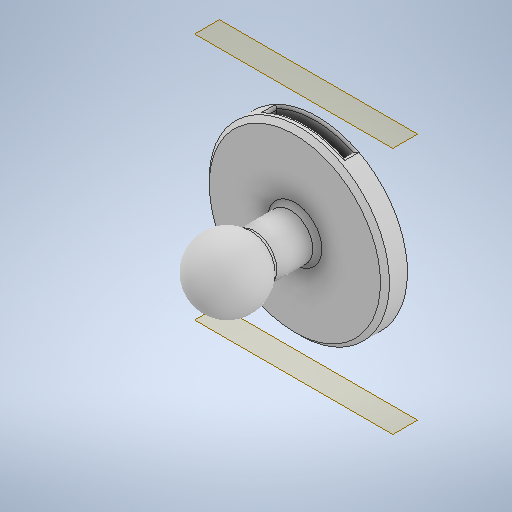
# Autodesk Inventor part: tagBase
Saved by Autodesk Inventor 2025 (Build 290162000, 162)
## iProperties
Created: 2026-08-22
Part Number: tagBase
Material: Generic
Document SubType Name: Modeling
Designer: PPSHS VR
Density: 1 g/cm^3
Appearance: Default
Author: PPSHS VR
Autodesk Inventor part; units mm, degrees
ref_plane "YZ Plane" through (0, 0, 0) normal (1, 0, 0) x (0, 1, 0)
ref_plane "XY Plane" through (0, 0, 0) normal (0, 0, 1) x (1, 0, 0)
sketch "Sketch1" plane through (0, 0, 0) normal (0, 0, 1) x (1, 0, 0)
  circle A0 centre (0, 0) radius 40
  dimension "d0" = 80
  constraints: 1 centre point, 1 coincident
  measures "d0" diameter of A0
extrude "Extrusion1" add sketch "Sketch1" along normal blind 10
chamfer "Chamfer1" distance 2 angle 45 1 edges at (-40, 0, 10)
ref_plane "Work Plane1" through (0, 55, 0) normal (0, 1, 0) x (-1, 0, 0)
sketch "Sketch3" plane through (0, 55, 0) normal (0, 1, 0) x (-1, 0, 0)
  line L0 (40, 0) -> (-40, 0) projected
  line L1 (40, 8) -> (-40, 8) projected
  line L2 (0, 0) -> (0, 1)
  line L3 (0, 1) -> (0, 3.25)
  line L4 (-17, 5.5) -> (17, 5.5)
  line L5 (17, 5.5) -> (17, 1)
  line L6 (17, 1) -> (-17, 1)
  line L7 (-17, 1) -> (-17, 5.5)
  line L8 (-17, 5.5) -> (17, 1) construction
  line L9 (17, 5.5) -> (-17, 1) construction
  dimension "d7" = 1
  dimension "d8" = 2.25
  dimension "d20" = 34
  constraints: 16 end point, 2 midpoint, 2 parallel, 2 vertical, 1 horizontal, 1 perpendicular
  measures "d7" distance of L2.start L2.end
  measures "d8" distance of L2.end L3.end
  measures "d20" distance of L5.end L6.end
extrude "Extrusion2" cut sketch "Sketch3" against normal blind 75
ref_plane "Work Plane2" through (0, -55, 0) normal (0, 1, 0) x (-1, 0, 0)
sketch "Sketch6" plane through (0, -55, 0) normal (0, 1, 0) x (-1, 0, 0)
  line L0 (40, 0) -> (-40, 0) projected
  line L1 (40, 8) -> (-40, 8) projected
  line L2 (0, 0) -> (0, 1)
  line L3 (0, 1) -> (0, 2)
  line L4 (17, 1) -> (-17, 1) projected
  line L5 (-6, 3) -> (6, 3)
  line L6 (6, 3) -> (6, 1)
  line L7 (6, 1) -> (-6, 1)
  line L8 (-6, 1) -> (-6, 3)
  line L9 (-6, 3) -> (6, 1) construction
  line L10 (6, 3) -> (-6, 1) construction
  dimension "d21" = 1
  dimension "d22" = 1
  dimension "d23" = 12
  constraints: 16 end point, 3 midpoint, 2 parallel, 2 point on line, 1 horizontal, 1 perpendicular, 1 vertical
  measures "d21" distance of L2.start L2.end
  measures "d22" distance of L2.end L3.end
  measures "d23" distance of L6.end L7.end
extrude "Extrusion4" cut sketch "Sketch6" along normal blind 65
sketch "Sketch8" plane through (0, 0, 10) normal (0, 0, 1) x (1, 0, 0)
  circle A0 centre (0, 0) radius 10
  dimension "d24" = 20
  constraints: 1 centre point, 1 coincident
  measures "d24" diameter of A0
extrude "Extrusion5" add sketch "Sketch8" along normal blind 30
sketch "Sketch9" plane through (0, 0, 40) normal (0, 0, 1) x (1, 0, 0)
  point P0 (0, 0)
sketch "Sketch10" plane through (0, 0, 0) normal (1, 0, 0) x (0, 1, 0)
  line L0 (10, 40) -> (-10, 40) projected
  arc A0 (15, 40) -> (-15, 40) centre (0, 40) ccw
  line L1 (15, 40) -> (-15, 40)
  point P0 (0, 0)
  dimension "d27" = 30
  constraints: 2 end point, 2 point on circle, 1 centre point, 1 horizontal, 1 midpoint
  measures "d27" diameter of A0
revolve "Revolution1" add sketch "Sketch10" angle 360 about axis through (0, 10, 40) along (0, -1, 0)
fillet "Fillet1" radius 2 2 edges at (-10, 0, 10) (-10, 0, 28.8197)
fillet "Fillet2" radius 1 4 edges at (0, 40, 5.5) (17, 36.2077, 3.25) (-17, 36.2077, 3.25) (0, 40, 1)
body "Solid1"
